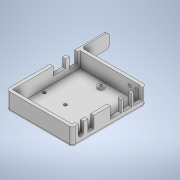
# Autodesk Inventor part: Part1
Saved by Autodesk Inventor 2022 (Build 260153000, 153)
## iProperties
Created: 2021-10-11
Part Number: Part1
Material: Generic
Document SubType Name: Modeling
Designer: Route
Density: 1 g/cm^3
Appearance: Default
Author: Route
Autodesk Inventor part; units mm, degrees
ref_plane "YZ Plane" through (0, 0, 0) normal (1, 0, 0) x (0, 1, 0)
ref_plane "XZ Plane" through (0, 0, 0) normal (0, 1, 0) x (-1, 0, 0)
ref_plane "XY Plane" through (0, 0, 0) normal (0, 0, 1) x (1, 0, 0)
sketch "Sketch1" plane through (0, 0, 0) normal (0, 1, 0) x (-1, 0, 0)
  line L0 (-30, -34) -> (30, -34)
  line L1 (30, -34) -> (30, 34)
  line L2 (30, 34) -> (-30, 34)
  line L3 (-30, 34) -> (-30, -34)
  line L4 (-30, -34) -> (30, 34) construction
  line L5 (30, -34) -> (-30, 34) construction
  line L6 (-33, 37) -> (33, 37)
  line L7 (33, 37) -> (33, -37)
  line L8 (33, -37) -> (-33, -37)
  line L9 (-33, -37) -> (-33, 37)
  line L10 (-33, 37) -> (33, -37) construction
  line L11 (33, 37) -> (-33, -37) construction
  point P0 (0, 0)
  dimension "d0" = 66
  dimension "d1" = 74
  constraints: 24 end point, 4 midpoint, 4 parallel, 2 horizontal, 2 perpendicular
  measures "d0" distance of L7.end L8.end
  measures "d1" distance of L6.end L7.end
extrude "Extrusion1" add sketch "Sketch1" along normal blind 3 contours L3 L2 L1 L0 | L6 L7 L8 L9
sketch "Sketch2" plane through (0, 3, 0) normal (0, 1, 0) x (1, 0, 0)
  line L0 (30, -34) -> (-30, -34)
  line L1 (-30, -34) -> (-30, 34)
  line L2 (-30, 34) -> (30, 34)
  line L3 (30, 34) -> (30, -34)
  line L4 (30, -34) -> (-30, 34) construction
  line L5 (-30, -34) -> (30, 34) construction
  line L6 (33, 37) -> (-33, 37) projected
  line L7 (33, -37) -> (-33, -37)
  line L8 (-33, -37) -> (-33, 37)
  line L9 (-33, 37) -> (33, 37)
  line L10 (33, 37) -> (33, -37)
  line L11 (33, -37) -> (-33, 37) construction
  line L12 (-33, -37) -> (33, 37) construction
  point P0 (0, 0)
  constraints: 24 end point, 4 midpoint, 4 parallel, 2 horizontal, 2 perpendicular
extrude "Extrusion2" add sketch "Sketch2" along normal blind 15
fillet "Fillet1" radius 3 4 edges at (33, 9, 37) (33, 9, -37) (-33, 9, -37) (-33, 9, 37)
fillet "Fillet2" radius 3 8 edges at (-32.1213, 0, 36.1213) (0, 0, 37) (32.1213, 0, 36.1213) (33, 0, 0) (32.1213, 0, -36.1213) (0, 0, -37) (-32.1213, 0, -36.1213) (-33, 0, 0)
sketch "Sketch3" plane through (0, 3, 0) normal (0, 1, 0) x (1, 0, 0)
  arc A0 (33, 34) -> (30, 37) centre (30, 34) ccw projected
  circle A1 centre (8.41, 30.19) radius 1.5
  line L0 (30, 37) -> (30, 34) projected
  circle A2 centre (26.19, 6.06) radius 1.5
  line L1 (-30, -34) -> (30, -34) projected
  circle A3 centre (-3.25, -27.65) radius 1.5
  circle A4 centre (8.41, 30.19) radius 3
  circle A5 centre (-3.25, -27.65) radius 3
  circle A6 centre (26.19, 6.06) radius 3
  point P0 (0, 0)
  dimension "d10" = 3
  dimension "d13" = 3
  dimension "d16" = 3
  dimension "d17" = 6
  dimension "d18" = 6
  dimension "d19" = 6
  constraints: 6 centre point, 3 coincident
  measures "d10" diameter of A1
  measures "d13" diameter of A2
  measures "d16" diameter of A3
  measures "d17" diameter of A4
  measures "d18" diameter of A5
  measures "d19" diameter of A6
extrude "Extrusion3" add sketch "Sketch3" along normal blind 2
sketch "Sketch4" plane through (0, 3, 0) normal (0, 1, 0) x (1, 0, 0)
  circle A0 centre (8.41, 30.19) radius 1.5 projected
  circle A1 centre (8.41, 30.19) radius 1.5
  circle A2 centre (26.19, 6.06) radius 1.5 projected
  circle A3 centre (26.19, 6.06) radius 1.5
  circle A4 centre (-3.25, -27.65) radius 1.5 projected
  circle A5 centre (-3.25, -27.65) radius 1.5
  point P0 (0, 0)
  constraints: 3 centre point, 3 coincident
extrude "Extrusion4" cut sketch "Sketch4" against normal blind 3
sketch "Sketch5" plane through (0, 0, 0) normal (0, -1, 0) x (1, 0, 0)
  circle A0 centre (8.41, -30.19) radius 1.5 projected
  circle A1 centre (8.41, -30.19) radius 3
  circle A2 centre (26.19, -6.06) radius 1.5 projected
  circle A3 centre (26.19, -6.06) radius 3
  circle A4 centre (-3.25, 27.65) radius 3 projected
  circle A5 centre (-3.25, 27.65) radius 3
  point P0 (0, 0)
  dimension "d24" = 6
  constraints: 3 centre point, 3 coincident
  measures "d24" diameter of A1
extrude "Extrusion5" cut sketch "Sketch5" against normal blind 2
sketch "Sketch6" plane through (-30, 3, 34) normal (1, 0, 0) x (0, 0, -1)
  line L0 (0, 0) -> (68, 0) projected
  line L1 (0, 0) -> (0, 3.6)
  line L2 (0, 15) -> (0, 0) projected
  line L3 (0, 15) -> (68, 15) projected
  line L4 (68, 0) -> (0, 0) projected
  line L5 (26.34, 6.8) -> (26.34, 15)
  line L6 (2.29, 4.35) -> (2.29, 15)
  line L7 (3.29, 3.6) -> (9.41, 3.6)
  line L8 (10.41, 4.35) -> (10.41, 15)
  line L9 (10.41, 4.35) -> (10.41, 5.45)
  line L10 (10.41, 4.35) -> (9.66, 3.6)
  line L11 (2.29, 4.35) -> (3.04, 3.6)
  line L12 (14.19, 6.8) -> (14.19, 15)
  line L13 (14.44, 6.8) -> (26.09, 6.8)
  line L14 (9.41, 3.6) -> (9.66, 3.6)
  line L15 (3.29, 3.6) -> (3.04, 3.6)
  line L16 (14.44, 6.8) -> (14.19, 6.8)
  line L17 (14.44, 6.8) -> (14.69, 6.8) construction
  line L18 (26.09, 6.8) -> (26.34, 6.8)
  line L19 (26.09, 6.8) -> (26.34, 6.8) construction
  point P0 (34, -3)
  point P1 (14.19, 15)
  point P2 (9.66, 3.6)
  point P3 (3.04, 3.6)
  point P4 (3.29, 3.6)
  point P5 (9.41, 3.6)
  dimension "d27" = 3.6
  dimension "d122" = 0.25
  dimension "d123" = 0.25
  dimension "d124" = 0.25
  dimension "d125" = 180
  dimension "d126" = 0.25
  dimension "d127" = 0
  constraints: 32 end point, 3 horizontal, 3 point on line, 2 collinear, 1 perpendicular
  measures "d27" distance of L0.start L1.end
  measures "d122" distance of L14.start L14.end
  measures "d123" distance of L15.start L15.end
  measures "d124" distance of L16.start L16.end
  measures "d125" angle of L16 L17
  measures "d126" distance of L18.start L18.end
  measures "d127" distance between parallel lines of L18 L19
sketch "Sketch7" plane through (30, 3, -34) normal (-1, 0, 0) x (0, 0, 1)
  line L0 (68, 0) -> (0, 0) projected
  line L1 (68, 0) -> (68, 3.6)
  line L2 (68, 0) -> (68, 15) projected
  line L3 (66.98, 3.6) -> (66.98, 6.14)
  line L4 (66.73, 3.6) -> (58.99, 3.6)
  line L5 (58.74, 3.6) -> (58.74, 6.14)
  line L6 (56.82, 3.6) -> (56.82, 6.14)
  line L7 (48.58, 6.14) -> (48.58, 3.6)
  line L8 (48.83, 3.6) -> (56.57, 3.6)
  line L9 (46.66, 3.6) -> (46.66, 6.14)
  line L10 (36, 6.14) -> (36, 3.6)
  line L11 (36.25, 3.6) -> (46.41, 3.6)
  line L12 (0, 15) -> (0, 0) projected
  line L13 (0, 0) -> (0, 15) projected
  line L14 (0, 3.6) -> (2.29, 3.6) construction
  arc A0 (2.89, 5.8) -> (7.89, 5.8) centre (5.39, 5.8) ccw
  line L15 (7.89, 5.8) -> (7.89, 15)
  line L16 (0, 15) -> (68, 15) projected
  line L17 (2.89, 5.8) -> (2.89, 15)
  line L18 (36, 6.14) -> (36, 15)
  line L19 (46.66, 6.14) -> (46.66, 15)
  line L20 (48.58, 6.14) -> (48.58, 15)
  line L21 (56.82, 6.14) -> (56.82, 15)
  line L22 (3.14, 15) -> (7.64, 15)
  line L23 (36.25, 15) -> (46.41, 15)
  line L24 (48.83, 15) -> (56.57, 15)
  line L25 (58.74, 6.14) -> (58.75, 15)
  line L26 (59, 15) -> (66.73, 15)
  line L27 (66.98, 6.14) -> (66.98, 15)
  line L28 (12.261, 3.6) -> (12.261, 15)
  line L29 (12.511, 3.6) -> (17.591, 3.6)
  line L30 (17.841, 3.6) -> (17.841, 15)
  line L31 (17.591, 3.6) -> (17.841, 3.6)
  line L32 (17.591, 3.6) -> (17.841, 3.6) construction
  line L33 (12.511, 3.6) -> (12.261, 3.6)
  line L34 (12.511, 3.6) -> (12.761, 3.6) construction
  line L35 (7.64, 5.8) -> (7.89, 5.8) construction
  line L36 (3.14, 5.8) -> (3.39, 5.8) construction
  line L37 (36.25, 3.6) -> (36, 3.6)
  line L38 (36.25, 3.6) -> (36.5, 3.6) construction
  line L39 (46.41, 3.6) -> (46.66, 3.6)
  line L40 (46.41, 3.6) -> (46.66, 3.6) construction
  line L41 (48.83, 3.6) -> (48.58, 3.6)
  line L42 (48.83, 3.6) -> (49.08, 3.6) construction
  line L43 (56.57, 3.6) -> (56.82, 3.6)
  line L44 (56.57, 3.6) -> (56.82, 3.6) construction
  line L45 (66.73, 3.6) -> (66.98, 3.6)
  line L46 (66.73, 3.6) -> (66.98, 3.6) construction
  line L47 (58.99, 3.6) -> (58.74, 3.6)
  line L48 (58.99, 3.6) -> (59.24, 3.6) construction
  line L49 (2.89, 15) -> (7.89, 15)
  line L50 (12.261, 15) -> (17.841, 15)
  line L51 (36, 15) -> (46.66, 15)
  line L52 (48.58, 15) -> (56.82, 15)
  line L53 (58.75, 15) -> (66.98, 15)
  point P0 (34, -3)
  point P1 (36, 15)
  point P2 (2.89, 5.8)
  point P3 (7.89, 5.8)
  point P4 (7.89, 15)
  point P5 (2.89, 15)
  point P6 (58.74, 3.6)
  point P7 (58.99, 3.6)
  point P8 (66.73, 3.6)
  point P9 (66.98, 3.6)
  point P10 (56.82, 3.6)
  point P11 (56.57, 3.6)
  point P12 (12.261, 15)
  dimension "d42" = 7.74
  dimension "d52" = 5
  dimension "d90" = 5.08
  dimension "d102" = 0.25
  dimension "d103" = 0
  dimension "d104" = 0.25
  dimension "d105" = 180
  dimension "d110" = 0.25
  dimension "d111" = 180
  dimension "d112" = 0.25
  dimension "d113" = 0
  dimension "d114" = 0.25
  dimension "d115" = 180
  dimension "d116" = 0.25
  dimension "d117" = 0
  dimension "d119" = 0
  dimension "d120" = 0.25
  dimension "d121" = 180
  constraints: 98 end point, 20 horizontal, 16 collinear, 5 perpendicular, 4 parallel, 3 vertical, 2 point on circle, 2 point on line, 1 centre point
  measures "d42" distance of L4.end L4.start
  measures "d52" diameter of A0
  measures "d90" distance of L29.start L29.end
  measures "d102" distance of L31.start L31.end
  measures "d103" distance between parallel lines of L31 L32
  measures "d104" distance of L33.start L33.end
  measures "d105" angle of L33 L34
  measures "d110" distance of L37.start L37.end
  measures "d111" angle of L37 L38
  measures "d112" distance of L39.start L39.end
  measures "d113" distance between parallel lines of L39 L40
  measures "d114" distance of L41.start L41.end
  measures "d115" angle of L41 L42
  measures "d116" distance of L43.start L43.end
  measures "d117" distance between parallel lines of L43 L44
  measures "d119" distance between parallel lines of L45 L46
  measures "d120" distance of L47.start L47.end
  measures "d121" angle of L47 L48
extrude "Extrusion6" cut sketch "Sketch7" against normal blind 3 contours L16 L15 A0 L17 | L27 L3 L45 L4 L47 L5 L25 L16 | L16 L30 L31 L29 L33 L28 | L21 L6 L43 L8 L41 L7 L20 L16 | L16 L19 L9 L39 L11 L37 L10 L18
extrude "Extrusion7" cut sketch "Sketch6" against normal blind 3
ref_plane "Work Plane1" through (30, 3, -1) normal (0, 0, -1) x (-1, 0, 0)
split body "Split1" result two bodies by plane through (30, 3, -1) normal (0, 0, -1) first body at (0.1787, 2.5, -11.4817)
move or copy body "Move Body1" bodies to move or copy 2 copy no translate (0, 0, 1.96)
combine bodies "Combine1" operation type add bodies to combine 3 2
ref_plane "Work Plane2" through (3, 3, 34) normal (1, 0, 0) x (0, 0, -1)
split body "Split2" result two bodies by plane through (3, 3, 34) normal (1, 0, 0) bodies 3 first body at (10.9943, 0.5, 1.619)
move or copy body "Move Body2" bodies to move or copy 4 copy no translate (-1.58, 0, 0)
combine bodies "Combine2" operation type add bodies to combine 4 5
mirror "Mirror1" about plane through (0, 0, 0) normal (0, 0, 1) remove original yes bodies 4
sketch "Sketch8" plane through (28.42, 3, -37) normal (0, 0, -1) x (-1, 0, 0)
  line L0 (61.42, 0) -> (58.42, 0) projected
  line L1 (58.42, 0) -> (29.21, 0)
  line L2 (0, 0) -> (-3, 0) projected
  line L3 (29.21, 0) -> (29.21, 15)
  line L4 (58.42, 15) -> (0, 15) projected
  line L5 (29.21, 0) -> (29.21, 12.8)
  line L6 (29.21, 12.8) -> (0, 12.8)
  line L7 (0, 15) -> (0, 3.6) projected
  line L8 (29.21, 15) -> (32.21, 15) construction
  line L9 (0, 15) -> (-3, 15) projected
  line L10 (29.21, 12.8) -> (13.21, 12.8)
  line L11 (13.21, 12.8) -> (13.21, 0)
  line L12 (0, 0) -> (58.42, 0) projected
  line L13 (29.21, 0) -> (32.21, 0)
  line L14 (32.21, 0) -> (32.21, 15)
  line L15 (0, 6.4) -> (13.21, 6.4)
  line L16 (6.605, 0) -> (6.605, 12.8)
  circle A0 centre (3.3025, 9.6) radius 1.5
  circle A1 centre (10, 9.6) radius 1.5
  point P0 (28.42, -3)
  dimension "d67" = 29.21
  dimension "d68" = 12.8
  dimension "d73" = 16
  dimension "d74" = 3
  dimension "d76" = 3
  dimension "d77" = 3
  constraints: 22 end point, 8 point on line, 4 perpendicular, 2 centre point, 2 midpoint, 1 collinear, 1 horizontal
  measures "d67" distance of L0.end L1.end
  measures "d68" distance of L1.end L5.end
  measures "d73" distance of L5.end L10.end
  measures "d74" distance of L1.end L13.end
  measures "d76" diameter of A0
  measures "d77" diameter of A1
extrude "Extrusion8" cut sketch "Sketch8" against normal blind 3 contours A0 | A1 bodies 4
sketch "Sketch9" plane through (28.42, 3, -37) normal (0, 0, -1) x (-1, 0, 0)
  line L0 (0, 15) -> (58.42, 15) projected
  line L1 (0, 15) -> (29.21, 15)
  line L2 (29.21, 15) -> (44.21, 15)
  line L3 (58.42, 15) -> (0, 15) projected
  line L4 (44.21, 15) -> (60.01, 15)
  line L5 (61.42, 15) -> (61.42, 0) projected
  line L6 (60.01, 15) -> (61.42, 15)
  line L7 (61.42, 15) -> (61.42, 1)
  line L8 (61.42, 1) -> (60.01, 1)
  line L9 (60.01, 1) -> (60.01, 15)
  point P0 (28.42, -3)
  dimension "d80" = 29.21
  dimension "d81" = 15
  dimension "d82" = 15.8
  dimension "d83" = 14
  constraints: 14 end point, 3 point on line, 2 parallel, 1 horizontal, 1 midpoint, 1 perpendicular
  measures "d80" distance of L0.start L1.end
  measures "d81" distance of L1.end L2.end
  measures "d82" distance of L2.end L4.end
  measures "d83" distance of L6.end L7.end
extrude "Extrusion9" add sketch "Sketch9" along normal mid plane 10 bodies 4
sketch "Sketch10" plane through (28.42, 3, -42) normal (0, 0, -1) x (-1, 0, 0)
  line L0 (61.42, 1) -> (61.42, 15) projected
  line L1 (60.01, 15) -> (58.42, 15) projected
  line L2 (61.42, 1) -> (60.01, 1)
  line L3 (60.01, 1) -> (60.01, 15)
  line L4 (60.01, 15) -> (61.42, 15)
  line L5 (61.42, 15) -> (61.42, 1)
  point P0 (28.42, -3)
  constraints: 8 end point, 2 parallel, 1 horizontal, 1 perpendicular
extrude "Extrusion10" add sketch "Sketch10" along normal blind 22 bodies 4
fillet "Fillet3" radius 3 3 edges at (-32.295, 18, -64) (-32.295, 4, -64) (-31.59, 11, -36.544)
sketch "Эскиз11" plane through (-30, 3, -34) normal (0, 1, 0) x (1, 0, 0)
  line L0 (58.42, -66.04) -> (0, -66.04) projected
  line L1 (58.42, -66.04) -> (20.878, -66.04)
  line L2 (58.42, -69.04) -> (0, -69.04) projected
  line L3 (20.878, -69.04) -> (54.813, -69.04) construction
  circle A0 centre (23.75, -38.094) radius 1.5
  circle A1 centre (3.123, -38.094) radius 1.5
  line L4 (-3, -66.04) -> (3.123, -66.04)
  line L5 (3.123, -66.04) -> (3.123, 3)
  line L6 (58.42, 3) -> (0, 3) projected
  line L7 (3.123, 3) -> (3.123, -38.094)
  line L8 (3.123, 3) -> (3.123, -38.094)
  point P0 (30, -34)
  dimension "d91" = 37.542
  dimension "d94" = 3
  dimension "d96" = 3
  dimension "d99" = 6.123
  dimension "d100" = 41.094
  dimension "d101" = 41.094
  constraints: 12 end point, 6 point on line, 2 centre point, 1 collinear, 1 horizontal, 1 vertical
  measures "d91" distance of L0.start L1.end
  measures "d94" diameter of A0
  measures "d96" diameter of A1
  measures "d99" distance of L4.start L4.end
  measures "d100" distance of L5.end L7.end
  measures "d101" distance of L5.end L7.end
extrude "Выдавливание11" cut sketch "Эскиз11" along normal mid plane 40 bodies 4
body "Solid4"
